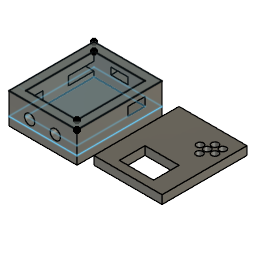
kraky (Autodesk Fusion 360 design; units mm, degrees)
Autodesk Fusion 360 part; units mm, degrees
sketch "Schizzo1" plane through (0, 0, 0) normal (0, 0, 1) x (1, 0, 0)
  line L0 (-20, 20) -> (40, 20)
  line L1 (40, 20) -> (40, -60)
  line L2 (40, -60) -> (-20, -60)
  line L3 (-20, -60) -> (-20, 20)
  constraint horizontal L0
  constraint vertical L1
  constraint horizontal L2
  constraint vertical L3
extrude "Estrusione1" add sketch "Schizzo1" along normal blind 5 makes body 1
delete_face "FacciaEliminazioneSuperficie1" leaving the opening 1 faces at (20, -60, 1.6667) on bodies 1
delete_face "FacciaEliminazioneSuperficie2" leaving the opening 1 faces at (40, -6.6667, 1.6667) on bodies 1
delete_face "FacciaEliminazioneSuperficie3" leaving the opening 1 faces at (0, -6.6667, 5) on bodies 1
delete_face "FacciaEliminazioneSuperficie4" leaving the opening 1 faces at (-20, -33.3333, 1.6667) on bodies 1
delete_face "FacciaEliminazioneSuperficie5" leaving the opening 1 faces at (0, 20, 1.6667) on bodies 1
delete_face "FacciaEliminazioneSuperficie6" leaving the opening 1 faces at (0, -6.6667, 0) on bodies 1
sketch "Schizzo2" plane through (0, 0, 0) normal (0, 0, 1) x (1, 0, 0)
  line L0 (-25, 25) -> (25, 25)
  line L1 (25, 25) -> (25, -40)
  line L2 (25, -40) -> (-25, -40)
  line L3 (-25, -40) -> (-25, 25)
  line L4 (-75, 25) -> (-50, 25)
  line L5 (-50, 25) -> (-50, -40)
  line L6 (-50, -40) -> (-75, -40)
  line L7 (-75, -40) -> (-75, 25)
  line L8 (50, 25) -> (75, 25)
  line L9 (75, 25) -> (75, -40)
  line L10 (75, -40) -> (50, -40)
  line L11 (50, -40) -> (50, 25)
  line L12 (-30, 50) -> (85, 50)
  line L13 (85, 50) -> (85, 75)
  line L14 (85, 75) -> (-30, 75)
  line L15 (-30, 75) -> (-30, 50)
  line L16 (-30, -65) -> (30, -65)
  line L17 (30, -65) -> (30, -90)
  line L18 (30, -90) -> (-30, -90)
  line L19 (-30, -90) -> (-30, -65)
  constraint horizontal L0
  constraint vertical L1
  constraint horizontal L2
  constraint vertical L3
  constraint horizontal L4
  constraint vertical L5
  constraint horizontal L6
  constraint vertical L7
  constraint horizontal L8
  constraint vertical L9
  constraint horizontal L10
  constraint vertical L11
  constraint horizontal L12
  constraint vertical L13
  constraint horizontal L14
  constraint vertical L15
  constraint horizontal L16
  constraint vertical L17
  constraint horizontal L18
  constraint vertical L19
sketch "Schizzo3" plane through (0, 0, 0) normal (0, 0, 1) x (1, 0, 0)
combine "Combina1" [no effect]
sketch "Schizzo4" plane through (0, 0, 0) normal (0, 1, 0) x (1, 0, 0)
sketch "Schizzo5" plane through (0, 0, 0) normal (0, 0, 1) x (1, 0, 0)
sketch "Schizzo6" plane through (0, 0, 0) normal (0, 0, 1) x (1, 0, 0)
  line L0 (90, -45) -> (30, -45)
  line L1 (30, -45) -> (30, 30)
  line L2 (30, 30) -> (90, 30)
  line L3 (90, 30) -> (90, -45)
  constraint horizontal L0
  constraint vertical L1
  constraint horizontal L2
  constraint vertical L3
combine "Combina2" [no effect]
sketch "Schizzo7" plane through (0, 0, 0) normal (0, 0, 1) x (1, 0, 0)
  line L0 (-20, 5) -> (20, 5)
  line L1 (20, 5) -> (20, -45)
  line L2 (20, -45) -> (-20, -45)
  line L3 (-20, -45) -> (-20, 5)
  line L4 (-15, 0) -> (15, 0)
  line L5 (15, 0) -> (15, -40)
  line L6 (15, -40) -> (-15, -40)
  line L7 (-15, -40) -> (-15, 0)
  constraint horizontal L0
  constraint vertical L1
  constraint horizontal L2
  constraint vertical L3
  constraint horizontal L4
  constraint vertical L5
  constraint horizontal L6
  constraint vertical L7
extrude "Estrusione4" add sketch "Schizzo7" along normal blind 5 separate body contours L0 L1 L2 L3 | L4 L5 L6 L7 makes body 2
extrude "Estrusione5" add sketch "Schizzo7" against normal blind 5 bodies 2
move_body "Sposta10" bodies 2 to x (-1, 0, 0) y (0, 1, 0) z (0, 0, -1) at (0, 0, 0)
extrude "Estrusione6" add 1 faces at (18.3333, -13.3333, 5) along direction (0, 0, 1) blind 5 on bodies 2 bodies 2
sketch "Schizzo8" plane through (0, 0, 10) normal (0, 0, 1) x (-1, 0, 0)
  line L0 (-15, 40) -> (15, 40)
  line L1 (15, 40) -> (15, 0)
  line L2 (15, 0) -> (-15, 0)
  line L3 (-15, 0) -> (-15, 40)
  line L4 (20, 45) -> (-20, 45)
  line L5 (-20, 45) -> (-20, -5)
  line L6 (-20, -5) -> (20, -5)
  line L7 (20, -5) -> (20, 45)
  line L8 (5, -5) -> (-5, -5)
  line L9 (-5, -5) -> (-5, 0)
  line L10 (-5, 0) -> (5, 0)
  line L11 (5, 0) -> (5, -5)
  constraint horizontal L8
  constraint vertical L9
  constraint horizontal L10
  constraint vertical L11
  constraint coincident L2 L9.end
  constraint coincident L6 L8.start
extrude "Estrusione7" cut sketch "Schizzo8" against normal blind 4 contours L2 L6 L8 L9 L10 L11 bodies 2
sketch "Schizzo9" plane through (0, 0, 0) normal (0, 0, 1) x (1, 0, 0)
sketch "Schizzo10" plane through (0, 0, 10) normal (0, 0, 1) x (-1, 0, 0)
  line L0 (5, 0) -> (5, -5)
  line L1 (5, -5) -> (20, -5)
  line L2 (20, -5) -> (20, 45)
  line L3 (20, 45) -> (-20, 45)
  line L4 (-20, 45) -> (-20, -5)
  line L5 (-20, -5) -> (-5, -5)
  line L6 (-5, -5) -> (-5, 0)
  line L7 (-5, 0) -> (-15, 0)
  line L8 (-15, 0) -> (-15, 40)
  line L9 (-15, 40) -> (15, 40)
  line L10 (15, 40) -> (15, 0)
  line L11 (15, 0) -> (5, 0)
  line L12 (-20, 15) -> (-15, 15)
  line L13 (-15, 15) -> (-15, 5)
  line L14 (-15, 5) -> (-20, 5)
  line L15 (-20, 5) -> (-20, 15)
  constraint horizontal L12
  constraint vertical L13
  constraint horizontal L14
  constraint vertical L15
  constraint coincident L8 L13.end
  constraint coincident L4 L12.start
extrude "Estrusione8" cut sketch "Schizzo10" against normal blind 5 contours L4 L8 L12 L13 L14 L15 bodies 2
sketch "Schizzo11" plane through (0, 0, 10) normal (0, 0, 1) x (-1, 0, 0)
  line L0 (-20, 15) -> (-15, 15)
  line L1 (-15, 15) -> (-15, 40)
  line L2 (-15, 40) -> (15, 40)
  line L3 (15, 40) -> (15, 0)
  line L4 (15, 0) -> (5, 0)
  line L5 (5, 0) -> (5, -5)
  line L6 (5, -5) -> (20, -5)
  line L7 (20, -5) -> (20, 45)
  line L8 (20, 45) -> (-20, 45)
  line L9 (-20, 45) -> (-20, 15)
  line L10 (-20, 45) -> (20, 45)
  line L11 (20, 45) -> (20, -5)
  line L12 (20, -5) -> (-20, -5)
  line L13 (-20, -5) -> (-20, 45)
  line L14 (-15, 40) -> (15, 40)
  line L15 (15, 40) -> (15, 0)
  line L16 (15, 0) -> (-15, 0)
  line L17 (-15, 0) -> (-15, 40)
  constraint horizontal L10
  constraint vertical L11
  constraint horizontal L12
  constraint vertical L13
  constraint coincident L6.end L7.start
  constraint coincident L8.end L9.start
  constraint horizontal L14
  constraint vertical L15
  constraint horizontal L16
  constraint vertical L17
  constraint coincident L3.end L4.start
  constraint coincident L1.end L2.start
extrude "Estrusione9" add sketch "Schizzo11" along normal blind 3 contours L0 L1 L2 L3 L4 L5 L6 L7 L8 L9 L10 L11 L12 L13 L14 L15 L16 L17 | L0 L5 L12 L13 L16 L17 bodies 2
hole "Foratura3" at (-7.828, -45, 4.4552) direction (0, 1, 0) diameter 6 depth 25 tip angle 180 bodies 2
hole "Foratura4" at (7.2521, -45, 4.2848) direction (0, 1, 0) diameter 6 depth 25 tip angle 180 bodies 2
sketch "Schizzo12" plane through (0, 0, 0) normal (0, 0, 1) x (1, 0, 0)
  line L0 (30, -45) -> (70, -45)
  line L1 (70, -45) -> (70, 5)
  line L2 (70, 5) -> (30, 5)
  line L3 (30, 5) -> (30, -45)
  line L4 (60, -40) -> (40, -40)
  line L5 (40, -40) -> (40, -25)
  line L6 (40, -25) -> (60, -25)
  line L7 (60, -25) -> (60, -40)
  constraint horizontal L0
  constraint vertical L1
  constraint horizontal L2
  constraint vertical L3
  constraint horizontal L4
  constraint vertical L5
  constraint horizontal L6
  constraint vertical L7
extrude "Estrusione10" add sketch "Schizzo12" along normal blind 5 separate body makes body 3
hole "Foratura5" at (59.9551, -12.9345, 5) direction (0, 0, -1) diameter 4 depth 25 tip angle 180 bodies 3
hole "Foratura6" at (60.0706, -8.4295, 5) direction (0, 0, -1) diameter 4 depth 25 tip angle 180 bodies 3
hole "Foratura7" at (60.0706, -3.9244, 5) direction (0, 0, -1) diameter 4 depth 25 tip angle 180 bodies 3
hole "Foratura8" at (64.5757, -8.4295, 5) direction (0, 0, -1) diameter 4 depth 25 tip angle 180 bodies 3
hole "Foratura9" at (55.7966, -8.4295, 5) direction (0, 0, -1) diameter 4 depth 25 tip angle 180 bodies 3
hole "Foratura10" at (64.5757, -3.8089, 5) direction (0, 0, -1) diameter 4 depth 25 tip angle 180 bodies 3
sketch "Schizzo13" plane through (0, 0, 13) normal (0, 0, 1) x (-1, 0, 0)
  line L0 (15, 0) -> (-15, 0)
  line L1 (-15, 0) -> (-15, 40)
  line L2 (-15, 40) -> (15, 40)
  line L3 (15, 40) -> (15, 0)
  line L4 (-20, -5) -> (20, -5)
  line L5 (20, -5) -> (20, 45)
  line L6 (20, 45) -> (-20, 45)
  line L7 (-20, 45) -> (-20, -5)
  line L8 (15, 40) -> (20, 40)
  line L9 (20, 40) -> (20, 30)
  line L10 (20, 30) -> (15, 30)
  line L11 (15, 30) -> (15, 40)
  constraint horizontal L8
  constraint vertical L9
  constraint horizontal L10
  constraint vertical L11
  constraint coincident L5 L9.end
  constraint coincident L2.end L3.start
extrude "Estrusione11" cut sketch "Schizzo13" against normal blind 10 contours L3 L5 L8 L9 L10 L11 bodies 2
sketch "Schizzo14" plane through (0, 0, 13) normal (0, 0, 1) x (-1, 0, 0)
  line L0 (20, 30) -> (15, 30)
  line L1 (15, 30) -> (15, 0)
  line L2 (15, 0) -> (-15, 0)
  line L3 (-15, 0) -> (-15, 40)
  line L4 (-15, 40) -> (20, 40)
  line L5 (20, 40) -> (20, 45)
  line L6 (20, 45) -> (-20, 45)
  line L7 (-20, 45) -> (-20, -5)
  line L8 (-20, -5) -> (20, -5)
  line L9 (20, -5) -> (20, 30)
  line L10 (-20, 45) -> (20, 45)
  line L11 (20, 45) -> (20, -5)
  line L12 (20, -5) -> (-20, -5)
  line L13 (-20, -5) -> (-20, 45)
  line L14 (-15, 40) -> (15, 40)
  line L15 (15, 40) -> (15, 0)
  line L16 (15, 0) -> (-15, 0)
  line L17 (-15, 0) -> (-15, 40)
  constraint horizontal L10
  constraint vertical L11
  constraint horizontal L12
  constraint vertical L13
  constraint coincident L8.end L9.start
  constraint coincident L6.end L7.start
  constraint horizontal L14
  constraint vertical L15
  constraint horizontal L16
  constraint vertical L17
  constraint coincident L1.end L2.start
  constraint coincident L3.end L4.start
sketch "Schizzo15" plane through (0, 0, 0) normal (0, 0, 1) x (1, 0, 0)
  line L0 (-35, -30) -> (-40, -30)
  line L1 (-40, -30) -> (-40, -20)
  line L2 (-40, -20) -> (-35, -20)
  line L3 (-35, -20) -> (-35, -30)
  constraint horizontal L0
  constraint vertical L1
  constraint horizontal L2
  constraint vertical L3
extrude "Estrusione12" add sketch "Schizzo15" along normal blind 5 separate body makes body 4
move_body "Sposta11" bodies 4 to x (1, 0, 0) y (0, 1, 0) z (0, 0, 1) at (20, -10, 8)
combine "Combina3" operation add target body 2 tool bodies 4
sketch "Schizzo16" plane through (0, 0, 13) normal (0, 0, 1) x (-1, 0, 0)
  line L0 (15, 0) -> (20, 0)
  line L1 (20, 0) -> (20, 15)
  line L2 (20, 15) -> (15, 15)
  line L3 (15, 15) -> (15, 0)
  constraint horizontal L0
  constraint vertical L1
  constraint horizontal L2
  constraint vertical L3
extrude "Estrusione13" cut sketch "Schizzo16" against normal blind 10 bodies 2
sketch "Schizzo17" plane through (0, 0, 0) normal (0, 0, 1) x (1, 0, 0)
  line L0 (-45, -5) -> (-40, -5)
  line L1 (-40, -5) -> (-40, -20)
  line L2 (-40, -20) -> (-45, -20)
  line L3 (-45, -20) -> (-45, -5)
  constraint horizontal L0
  constraint vertical L1
  constraint horizontal L2
  constraint vertical L3
extrude "Estrusione14" add sketch "Schizzo17" along normal blind 5 separate body makes body 5
move_body "Sposta12" bodies 5 to x (1, 0, 0) y (0, 1, 0) z (0, 0, 1) at (25, 5, 8)
combine "Combina4" operation add target body 5 tool bodies 2
